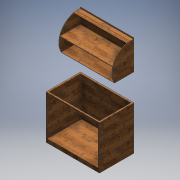
# Autodesk Inventor part: esqueleto_mueble
Saved by Autodesk Inventor 2016 (Build 200138000, 138)
## iProperties
Created: 2015-11-24
Part Number: esqueleto_mueble
Material: Lead
Document SubType Name: Modeling
Designer: Daniela
Density: 11.34 g/cm^3
Appearance: Glossy - Black
Author: Daniela
Autodesk Inventor part; units mm, degrees
ref_plane "YZ Plane" through (0, 0, 0) normal (1, 0, 0) x (0, 1, 0)
ref_plane "XZ Plane" through (0, 0, 0) normal (0, 1, 0) x (-1, 0, 0)
ref_plane "XY Plane" through (0, 0, 0) normal (0, 0, 1) x (1, 0, 0)
sketch "Sketch1" plane through (0, 0, 0) normal (0, 0, 1) x (1, 0, 0)
  line L0 (0, 0) -> (1100, 0)
  line L1 (1100, 0) -> (1100, 10)
  line L2 (1100, 10) -> (0, 10)
  line L3 (0, 10) -> (0, 0)
  dimension "ancho" = 1100
  dimension "espesor" = 10
  constraints: 8 end point, 2 parallel, 1 horizontal, 1 perpendicular
  measures "ancho" distance of L1.end L2.end
  measures "espesor" distance of L0.end L1.end
extrude "Extrusion1" add sketch "Sketch1" along normal blind 900
sketch "Sketch2" plane through (0, 0, 0) normal (0, -1, 0) x (1, 0, 0)
  line L0 (0, 0) -> (1100, 0) construction
  line L1 (1100, 0) -> (1100, 900) construction
  line L2 (0, 900) -> (1100, 900) construction
  line L3 (0, 0) -> (0, 900) construction
  line L4 (0, 0) -> (0, 900) projected
  line L5 (0, 70) -> (1100, 70)
  line L6 (1100, 70) -> (1100, 80)
  line L7 (1100, 80) -> (0, 80)
  line L8 (0, 80) -> (0, 70)
  line L9 (0, 900) -> (1100, 900) projected
  line L10 (1100, 0) -> (1100, 900) projected
  line L11 (0, 900) -> (1100, 900)
  line L12 (1100, 900) -> (1100, 890)
  line L13 (1100, 890) -> (0, 890)
  line L14 (0, 890) -> (0, 900)
  dimension "d5" = 10
  dimension "d6" = 10
  dimension "d7" = 80
  constraints: 16 end point, 4 parallel, 3 point on line, 2 horizontal, 2 perpendicular
  measures "d5" distance between parallel lines of L5 L7
  measures "d6" distance between parallel lines of L2 L13
  measures "d7" distance between parallel lines of L0 L7
extrude "Extrusion2" add sketch "Sketch2" along normal blind 700 contours L4 L7 L6 L5 | L4 L9 L10 L13
sketch "Sketch3" plane through (0, 0, 900) normal (0, 0, 1) x (1, 0, 0)
  line L0 (1100, 10) -> (1100, -700) projected
  line L1 (1100, 10) -> (0, 10) projected
  line L2 (0, 10) -> (0, -700) projected
  line L3 (1100, -700) -> (0, -700) projected
  line L4 (30, -670) -> (30, -20)
  line L5 (30, -20) -> (1070, -20)
  line L6 (1070, -20) -> (1070, -670)
  line L7 (1070, -670) -> (30, -670)
  point P0 (0, 0)
  dimension "d10" = 30
  constraints: 8 end point, 3 other
  measures "d10" distance between parallel lines of L1 L5
extrude "Extrusion3" cut sketch "Sketch3" against normal up to next contours L4 L5 L6 L7
sketch "Sketch4" plane through (0, -700, 0) normal (0, -1, 0) x (1, 0, 0)
  line L0 (0, 70) -> (1100, 70) construction
  line L1 (1100, 70) -> (1100, 80) construction
  line L2 (1100, 80) -> (0, 80) construction
  line L3 (0, 80) -> (0, 70) construction
  line L4 (0, 900) -> (0, 890) construction
  line L5 (0, 890) -> (1100, 890) construction
  line L6 (1100, 890) -> (1100, 900) construction
  line L7 (1100, 900) -> (0, 900) construction
  line L8 (1100, 70) -> (0, 70) construction
  line L9 (0, 0) -> (0, 70) construction
  line L10 (0, 0) -> (1100, 0) construction
  line L11 (1100, 0) -> (1100, 70) construction
  line L12 (0, 900) -> (1100, 900)
  line L13 (1100, 900) -> (1100, 0)
  line L14 (1100, 0) -> (0, 0)
  line L15 (0, 0) -> (0, 900)
  line L16 (1100, 80) -> (0, 80) projected
  line L17 (30, 80) -> (1070, 80)
  line L18 (1070, 80) -> (1070, 890)
  line L19 (1070, 890) -> (30, 890)
  line L20 (30, 890) -> (30, 80)
  dimension "d13" = 30
  dimension "d14" = 30
  constraints: 16 end point, 4 parallel, 2 horizontal, 2 perpendicular, 2 point on line
  measures "d13" distance between parallel lines of L15 L20
  measures "d14" distance between parallel lines of L18 L13
extrude "Extrusion4" add sketch "Sketch4" against normal blind 10 contours L12 L13 L16 L18 L19 L20 L15 | L16 L13 L14 L15
ref_plane "Work Plane1" through (0, 0, 1450) normal (0, 0, 1) x (1, 0, 0)
sketch "Sketch5" plane through (0, 0, 1450) normal (0, 0, 1) x (1, 0, 0)
  line L0 (1100, 10) -> (0, 10) projected
  line L1 (0, 10) -> (0, -700) projected
  line L2 (1100, 10) -> (1100, -700) projected
  line L3 (1100, -700) -> (0, -700) projected
  point P0 (0, 0)
extrude "Extrusion5" add sketch "Sketch5" along normal blind 10
sketch "Sketch6" plane through (0, 0, 1460) normal (0, 0, 1) x (1, 0, 0)
  line L0 (1100, 10) -> (0, 10) projected
  line L1 (0, 10) -> (0, -700) projected
  line L2 (0, -700) -> (1100, -700) projected
  line L3 (1100, -700) -> (1100, 10) projected
  line L4 (1100, -700) -> (0, -700) projected
  line L5 (1100, 0) -> (1100, -690) projected
  line L6 (0, -700) -> (1100, -700)
  line L7 (1100, -700) -> (1100, -690)
  line L8 (1100, -690) -> (0, -690)
  line L9 (0, -690) -> (0, -700)
  line L10 (0, 0) -> (0, -690) projected
  line L11 (1100, 10) -> (0, 10)
  line L12 (0, 10) -> (0, 0)
  line L13 (0, 0) -> (1100, 0)
  line L14 (1100, 0) -> (1100, 10)
  dimension "d20" = 10
  dimension "d21" = 10
  constraints: 16 end point, 4 parallel, 2 horizontal, 2 perpendicular, 2 point on line
  measures "d20" distance between parallel lines of L2 L8
  measures "d21" distance between parallel lines of L0 L13
extrude "Extrusion6" add sketch "Sketch6" along normal blind 580 contours L3 L13 L1 L0 | L3 L2 L1 L8
sketch "Sketch7" plane through (0, -700, 1450) normal (0, -1, 0) x (1, 0, 0)
  line L0 (1100, 0) -> (1100, 590) projected
  line L1 (0, 590) -> (1100, 590) projected
  line L2 (0, 0) -> (0, 590) projected
  line L3 (0, 10) -> (1100, 10) projected
  line L4 (30, 10) -> (1070, 10)
  line L5 (1070, 10) -> (1070, 560)
  line L6 (1070, 560) -> (30, 560)
  line L7 (30, 560) -> (30, 10)
  line L8 (0, 0) -> (1100, 0) projected
  point P0 (0, -1450)
  dimension "d24" = 30
  dimension "d25" = 30
  dimension "d26" = 30
  constraints: 8 end point, 2 parallel, 1 horizontal, 1 perpendicular, 1 point on line
  measures "d24" distance between parallel lines of L2 L7
  measures "d25" distance between parallel lines of L5 L0
  measures "d26" distance between parallel lines of L1 L6
extrude "Extrusion7" cut sketch "Sketch7" against normal up to next contours L3 L7 L6 L5
sketch "Sketch9" plane through (0, -700, 0) normal (0, -1, 0) x (1, 0, 0)
  line L0 (0, 900) -> (0, 0) construction
  line L1 (1100, 900) -> (1100, 0) construction
  line L2 (1100, 890) -> (1100, 80) projected
  line L3 (0, 900) -> (1100, 900)
  line L4 (1100, 900) -> (1100, 870)
  line L5 (1100, 870) -> (0, 870)
  line L6 (0, 870) -> (0, 900)
  line L7 (1100, 0) -> (0, 0) projected
  line L8 (1100, 900) -> (0, 900) projected
  constraints: 8 end point, 2 parallel, 1 horizontal, 1 perpendicular, 1 point on line
extrude "Extrusion9" add sketch "Sketch9" against normal blind 10
ref_plane "Work Plane2" through (0, 0, 1740) normal (0, 0, 1) x (1, 0, 0)
sketch "Sketch12" plane through (0, 0, 1740) normal (0, 0, 1) x (1, 0, 0)
  line L0 (1100, -690) -> (1100, 0) projected
  line L1 (1100, 0) -> (0, 0) projected
  line L2 (0, -690) -> (1100, -690) projected
  line L3 (0, -690) -> (0, 0) projected
  point P0 (0, 0)
extrude "Extrusion11" add sketch "Sketch12" along normal blind 10
sketch "Sketch14" plane through (1100, 0, 890) normal (0, 0, -1) x (-1, 0, 0)
  line L0 (0, 0) -> (0, -690) projected
  line L1 (0, 0) -> (30, 0)
  line L2 (30, 0) -> (30, -690)
  line L3 (30, -690) -> (0, -690)
  line L4 (0, -690) -> (0, 0)
  line L5 (0, -690) -> (1100, -690) projected
  line L6 (0, 0) -> (1100, 0) projected
  line L7 (1100, -690) -> (1070, -690)
  line L8 (1070, -690) -> (1070, 0)
  line L9 (1070, 0) -> (1100, 0)
  line L10 (1100, 0) -> (1100, -690)
  constraints: 16 end point, 4 parallel, 2 horizontal, 2 perpendicular, 1 point on line
extrude "Extrusion13" add sketch "Sketch14" along normal blind 890 contours L1 L2 L3 L0 | L6 L10 L5 L8
ref_plane "Work Plane3" through (0, 0, 2010) normal (0, 0, 1) x (1, 0, 0)
sketch "Sketch15" plane through (0, 0, 2010) normal (0, 0, 1) x (1, 0, 0)
  line L0 (0, -690) -> (0, -700) projected
  line L1 (0, -690) -> (1100, -690)
  line L2 (1100, -690) -> (1100, 0)
  line L3 (1100, 0) -> (0, 0)
  line L4 (0, 0) -> (0, -690)
  point P0 (0, 0)
  constraints: 8 end point, 2 parallel, 1 horizontal, 1 perpendicular
extrude "Extrusion14" add sketch "Sketch15" along normal blind 10
sketch "Sketch16" plane through (0, 0, 2020) normal (0, 0, 1) x (1, 0, 0)
  line L0 (0, 10) -> (0, -700) projected
  line L1 (0, -700) -> (10, -700)
  line L2 (10, -700) -> (10, 10)
  line L3 (10, 10) -> (0, 10)
  line L4 (0, 10) -> (0, -700)
  line L5 (1100, -700) -> (0, -700) projected
  line L6 (1100, 10) -> (0, 10) projected
  line L7 (1100, -700) -> (1090, -700)
  line L8 (1090, -700) -> (1090, 10)
  line L9 (1090, 10) -> (1100, 10)
  line L10 (1100, 10) -> (1100, -700)
  point P0 (0, 0)
  dimension "d57" = 10
  dimension "d58" = 10
  constraints: 16 end point, 4 parallel, 2 horizontal, 2 perpendicular, 1 point on line
  measures "d57" distance between parallel lines of L0 L2
  measures "d58" distance between parallel lines of L10 L8
extrude "Extrusion15" add sketch "Sketch16" against normal up to surface (570 mm away) contours L3 L2 L1 L0 | L6 L10 L5 L8
sketch "Sketch17" plane through (1100, -700, 1450) normal (1, 0, 0) x (0, 0, -1)
  line L0 (-300, 10) -> (-300, 700) projected
  line L1 (0, 710) -> (-590, 710) projected
  line L2 (-590, 700) -> (-590, 710) projected
  line L3 (-570, 700) -> (-590, 700) projected
  line L4 (-570, 10) -> (-570, 700) projected
  line L5 (-570, 10) -> (-590, 10) projected
  line L6 (-590, 0) -> (-590, 10) projected
  line L7 (0, 0) -> (-590, 0) projected
  line L8 (0, 0) -> (0, 710) projected
  line L9 (0, 710) -> (0, 310)
  line L10 (0, 0) -> (0, 710) projected
  arc A0 (-570, 700) -> (0, 310) centre (-171.0094, 671.6017) ccw
  point P0 (1450, 700)
  dimension "d61" = 400
  dimension "d62" = 400
  constraints: 2 end point, 2 point on circle, 1 centre point, 1 point on line
  measures "d61" distance of L1.start L9.end
  measures "d62" radius of A0
extrude "Extrusion16" cut sketch "Sketch17" against normal up to next contours L8 L7 L6 L5 L4 A0
equation "\"d5\" = espesor"
equation "\"d6\" = espesor"
equation "\"d10\" = 3 * espesor"
equation "\"d13\" = 3 * espesor"
equation "\"d14\" = 3 * espesor"
equation "\"d15\" = espesor"
equation "\"d18\" = espesor"
equation "\"d20\" = espesor"
equation "\"d21\" = espesor"
equation "\"d24\" = 3 * espesor"
equation "\"d25\" = 3 * espesor"
equation "\"d26\" = 3 * espesor"
equation "\"d33\" = espesor"
equation "\"d41\" = espesor"
equation "\"d47\" = h_inf - espesor"
equation "\"d55\" = espesor"
equation "\"d57\" = espesor"
equation "\"d58\" = espesor"
equation "\"d59\" = espesor"
equation "\"d63\" = espesor"
equation "\"h_inf\" = 900"
body "Solid1"
